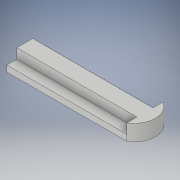
# Autodesk Inventor part: tenshoner slider
Saved by Autodesk Inventor 2019 (Build 230136000, 136)
## iProperties
Created: 2019-12-07
Part Number: tenshoner slider
Material: Generic
Document SubType Name: Modeling
Designer: User
Density: 1 g/cm^3
Appearance: Default
Author: User
Autodesk Inventor part; units mm, degrees
ref_plane "YZ Plane" through (0, 0, 0) normal (1, 0, 0) x (0, 1, 0)
ref_plane "XZ Plane" through (0, 0, 0) normal (0, 1, 0) x (-1, 0, 0)
ref_plane "XY Plane" through (0, 0, 0) normal (0, 0, 1) x (1, 0, 0)
sketch "Sketch1" plane through (0, 0, 0) normal (1, 0, 0) x (0, 1, 0)
  line L0 (0, 0) -> (0.9652, 0)
  line L1 (0.9652, 0) -> (0.9652, -5.715)
  line L2 (0.9652, -5.715) -> (0, -5.715)
  line L3 (0, -5.715) -> (0, 0)
  line L4 (0.9652, -1.5875) -> (2.54, -1.5875)
  line L5 (2.54, -1.5875) -> (2.54, -4.1275)
  line L6 (2.54, -4.1275) -> (0.9652, -4.1275)
  line L7 (0.9652, -4.1275) -> (0.9652, -1.5875)
  dimension "d0" = 5.715
  dimension "d1" = 2.54
  dimension "d2" = 1.5875
  dimension "d3" = 0.9652
  dimension "d4" = 1.5748
  constraints: 16 end point, 4 parallel, 2 horizontal, 2 perpendicular, 1 point on line
  measures "d0" distance of L2.end L0.start
  measures "d1" distance between parallel lines of L6 L4
  measures "d2" distance between parallel lines of L2 L6
  measures "d3" distance between parallel lines of L3 L1
  measures "d4" distance between parallel lines of L1 L5
extrude "Extrusion1" add sketch "Sketch1" along normal blind 19.05
sketch "Sketch2" plane through (0, 0, -5.715) normal (0, -1, 0) x (1, 0, 0)
  line L0 (19.05, 5.715) -> (19.05, 0) projected
  arc A0 (19.05, 0) -> (19.05, 5.715) centre (17.3414, 2.8575) ccw
  point P0 (0, 5.715)
  constraints: 2 point on circle, 1 centre point
extrude "Extrusion2" add sketch "Sketch2" against normal up to surface (2.54 mm away)
equation "\"d2\" = -0.5 * d1 + 0.5 * d0"
body "Solid1"
